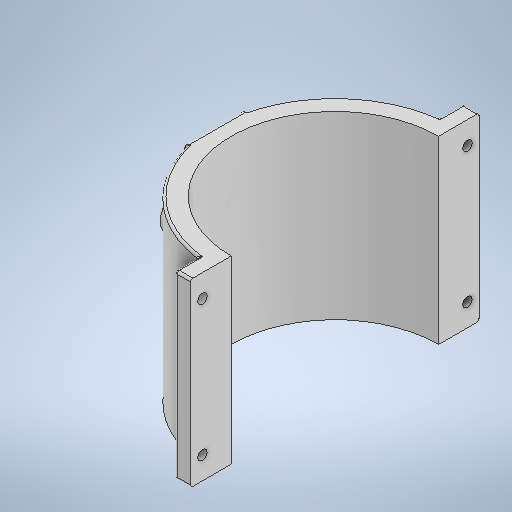
# Autodesk Inventor part: motor-mount
Saved by Autodesk Inventor 2025.2 (Build 292293000, 293)
## iProperties
Created: 2025-02-07
Part Number: motor-mount
Material: 一般
Document SubType Name: Modeling
Designer: mahhy
Density: 1 g/cm^3
Appearance: 既定
Author: mahhy
## iProperties of the stored document motor-mount_3D プリント.ipt
Created: 2025-02-10
Part Number: motor-mount_3D プリント
Material: 一般
Document SubType Name: Modeling
Designer: mahhy
Density: 1 g/cm^3
Appearance: 既定
Author: mahhy
Autodesk Inventor part; units mm, degrees
ref_plane "YZ Plane" through (0, 0, 0) normal (1, 0, 0) x (0, 1, 0)
ref_plane "XZ Plane" through (0, 0, 0) normal (0, 1, 0) x (-1, 0, 0)
ref_plane "XY Plane" through (0, 0, 0) normal (0, 0, 1) x (1, 0, 0)
sketch "スケッチ1" plane through (0, 0, 0) normal (0, 1, 0) x (-1, 0, 0)
  line L0 (0, 0) -> (60, 0)
  line L1 (60, 0) -> (60, -120)
  line L2 (60, -120) -> (0, -120)
  line L3 (0, -120) -> (0, 0)
  circle A0 centre (0, -60) radius 46
  circle A1 centre (0, -60) radius 54
  line L4 (0, -14) -> (7, -14)
  line L5 (7, -14) -> (7, 4)
  line L6 (7, 4) -> (0, 4)
  line L7 (0, 4) -> (0, -14)
  line L8 (0, -106) -> (7, -106)
  line L9 (7, -106) -> (7, -124)
  line L10 (7, -124) -> (0, -124)
  line L11 (0, -124) -> (0, -106)
  line L12 (54, -47.5) -> (46, -47.5)
  line L13 (46, -47.5) -> (46, -72.5)
  line L14 (46, -72.5) -> (54, -72.5)
  line L15 (54, -72.5) -> (54, -47.5)
  point P0 (46, -60)
  point P1 (46, -60)
  point P2 (7, -113.5444)
  point P3 (52.5333, -72.5)
  point P4 (52.5333, -47.5)
  point P5 (7, -6.4556)
  point P6 (7, 0)
  dimension "d0" = 60
  dimension "d1" = 120
  dimension "d2" = 92
  dimension "d3" = 108
  dimension "d4" = 7
  dimension "d5" = 18
  dimension "d6" = 7
  dimension "d7" = 18
  dimension "d8" = 8
  dimension "d9" = 25
  dimension "d11" = 0
  dimension "d12" = 0
  constraints: 32 end point, 8 parallel, 4 horizontal, 4 perpendicular, 3 point on circle, 2 centre point, 2 midpoint, 2 point on line, 1 coincident
  measures "d0" distance of L1.end L2.end
  measures "d1" distance of L0.end L1.end
  measures "d2" diameter of A0
  measures "d3" diameter of A1
  measures "d4" distance of L6.end L5.end
  measures "d5" distance of L5.end L4.end
  measures "d6" distance of L9.end L10.end
  measures "d7" distance of L8.end L9.end
  measures "d8" distance of L14.end L13.end
  measures "d9" distance of L13.end L12.end
  measures "d11" vertical distance of A0.centre point (46, -60)
  measures "d12" distance of point (46, -60) point (46, -60)
extrude "押し出し1" add sketch "スケッチ1" along normal blind 80 contours L7 L6 L5 L0 | L0 L5 A1 L3 | A1 L5 L4 L3 | A1 L12 L13 A0 L4 L5 | A1 L9 L2 L3 | L3 L8 L9 A1 | L12 L15 A1 | A1 L14 L13 L12 | A0 L13 L14 A1 L9 L8 | L2 L9 L10 L11 | L15 L14 A1
sketch "スケッチ2" plane through (-54, 0, -72.5) normal (-1, 0, 0) x (0, 0, 1)
  line L0 (-33.5, 0) -> (58.5, 0) projected
  line L1 (0, 0) -> (0, 80) projected
  circle A0 centre (12.5, 40) radius 12.5
  point P0 (72.5, 0)
  point P1 (12.5, 0)
  point P2 (0, 40)
  point P3 (0, 40)
  dimension "d15" = 0
  dimension "d17" = 25
  constraints: 3 midpoint, 1 centre point, 1 coincident, 1 horizontal alignment
  measures "d15" horizontal distance of point (12.5, 0) point (12.5, 40)
  measures "d17" diameter of A0
extrude "押し出し2" add sketch "スケッチ2" along normal blind 1
sketch "スケッチ3" plane through (-55, 40, -60) normal (-1, 0, 0) x (0, 0, 1)
  circle A0 centre (0, 0) radius 8.5
  circle A1 centre (0, 0) radius 12.5 projected
  point P0 (60, -40)
  dimension "d20" = 17
  constraints: 1 centre point, 1 concentric
  measures "d20" diameter of A0
extrude "押し出し3" add sketch "スケッチ3" along normal blind 15 contours A0
sketch "スケッチ4" plane through (-7, 0, -124) normal (-1, 0, 0) x (0, 0, 1)
  line L0 (0, 80) -> (10.4556, 80) projected
  line L1 (0, 0) -> (10.4556, 0) projected
  line L2 (117.5444, 80) -> (128, 80) projected
  line L3 (117.5444, 0) -> (124, 0) projected
  point P0 (5.2278, 70)
  point P1 (5.2278, 10)
  point P2 (122.7722, 10)
  point P3 (5.2278, 80)
  point P4 (5.2278, 0)
  point P5 (120.7722, 0)
  point P6 (122.7722, 70)
  point P7 (122.7722, 80)
  dimension "d23" = 0
  dimension "d24" = 10
  dimension "d25" = 0
  dimension "d26" = 10
  dimension "d28" = 10
  dimension "d36" = 0
  dimension "d37" = 10
  constraints: 4 midpoint
  measures "d23" horizontal distance of point (5.228, 80) point (5.228, 70)
  measures "d24" distance from line of L0 point (5.228, 70)
  measures "d25" horizontal distance of point (5.228, 0) point (5.228, 10)
  measures "d26" distance from line of L1 point (5.228, 10)
  measures "d28" vertical distance of point (120.772, 0) point (122.772, 10)
  measures "d36" horizontal distance of point (122.772, 80) point (122.772, 70)
  measures "d37" distance from line of L2 point (122.772, 70)
hole "穴1" at (-7, 70, -118.7722) at (-7, 10, -118.7722) at (-7, 10, -1.2278) at (-7, 70, -1.2278) direction (1, 0, 0) diameter 4.2 end through all
fillet "フィレット1" radius 1 12 edges at (-3.5, 80, -124) (-3.5, 80, 4) (-7, 80, -1.2278) (-7, 80, -118.7722) (-36.1554, 80, -100.1097) (-36.1554, 80, -19.8903) (-7, 40, 4) (-36.1554, 0, -19.8903) (-3.5, 0, 4) (-36.1554, 0, -100.1097) (-3.5, 0, -124) (-7, 0, -118.7722)
fillet "フィレット2" radius 2 2 edges at (-54, 80, -60) (-54, 0, -60)
fillet "フィレット3" radius 1 2 edges at (-55, 40, -72.5) (-70, 40, -68.5)
fillet "フィレット4" radius 1 5 edges at (-6.669, 79.7433, -113.253) (-6.669, 0.2567, -113.253) (-7, 40, -113.5444) (-6.669, 79.7433, -6.747) (-7, 40, -6.4556)
